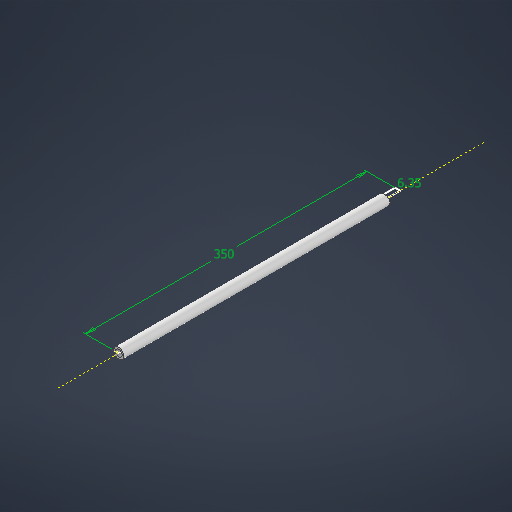
# Autodesk Inventor part: Suspenion_Arm_Assembly_V2_Member
Saved by Autodesk Inventor 2027 (Build 310192000, 192)
## iProperties
Created: 2026-09-20
Part Number: Suspenion_Arm_Assembly_V2_Member
Material: Generic
Document SubType Name: Modeling
Designer: share
Density: 1 g/cm^3
Appearance: Default
Density: 7.85 g/cm^3
Appearance: Semi-Polished
Mass: 289.986 g
Surface Area: 141.452 cm^2
Volume: 36.9409 cm^3
Author: share
Autodesk Inventor part; units mm, degrees
ref_plane "YZ Plane" through (0, 0, 0) normal (1, 0, 0) x (0, 1, 0)
ref_plane "XZ Plane" through (0, 0, 0) normal (0, 1, 0) x (-1, 0, 0)
ref_plane "XY Plane" through (0, 0, 0) normal (0, 0, 1) x (1, 0, 0)
sketch "Sketch1" plane through (0, 0, 0) normal (0, 1, 0) x (-1, 0, 0)
  line L0 (0, -456) -> (0, 76) construction
  line L1 (-1.27, 0) -> (7.62, 0) construction
  line L2 (0, 0) -> (6.35, 0)
  line L3 (6.35, 0) -> (6.35, -350)
  line L4 (6.35, -350) -> (0, -350)
  line L5 (0, -350) -> (0, 0)
  dimension "d0" = 350
  dimension "d1" = 6.35
  constraints: 8 end point, 2 parallel, 1 horizontal, 1 perpendicular
  measures "d0" distance between parallel lines of L4 L1
  measures "d1" distance between parallel lines of L5 L3
revolve "Revolution1" add sketch "Sketch1" angle 360 about axis through (0, 0, -350) along (0, 0, 1)
sketch "Sketch2" plane through (0, 0, 0) normal (0, 1, 0) x (-1, 0, 0)
  line L0 (6.35, -350) -> (-6.35, -350) projected
  circle A0 centre (0, -350) radius 20
  point P0 (0, 0)
  dimension "d3" = 40
  constraints: 1 centre point, 1 midpoint
  measures "d3" diameter of A0
extrude "Extrusion1" cut sketch "Sketch2" along normal through all both and the other way through all
sketch "Sketch3" plane through (0, 0, 0) normal (0, 0, 1) x (1, 0, 0)
  circle A0 centre (0, 0) radius 4.2164
  point P0 (0, 0)
  dimension "d6" = 8.4328
  constraints: 1 centre point, 1 coincident
  measures "d6" diameter of A0
extrude "Extrusion2" cut sketch "Sketch3" against normal blind 50.8
thread "Thread1" size "3/8-24 UNF" class "2B" standard "ANSI Unified Screw Threads" full length
body "Solid1"
